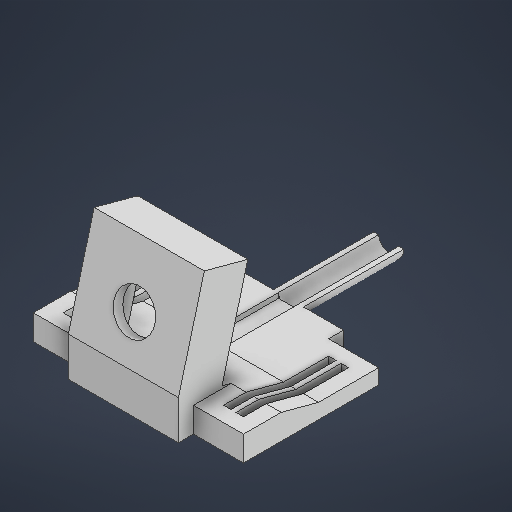
# Autodesk Inventor part: pieza prueba autodesk
Saved by Autodesk Inventor 2027.1 (Build 311270010, 270A)
## iProperties
Created: 2026-09-10
Part Number: pieza prueba autodesk
Material: Genérico
Document SubType Name: Modeling
Designer: marco
Density: 1 g/cm^3
Appearance: Valor por defecto
Author: marco
Autodesk Inventor part; units mm, degrees
ref_plane "YZ Plane" through (0, 0, 0) normal (1, 0, 0) x (0, 1, 0)
ref_plane "XZ Plane" through (0, 0, 0) normal (0, 1, 0) x (-1, 0, 0)
ref_plane "XY Plane" through (0, 0, 0) normal (0, 0, 1) x (1, 0, 0)
sketch "Boceto9" plane through (0, 0, 0) normal (1, 0, 0) x (0, 1, 0)
  line L0 (0, 0) -> (0, -3)
  line L1 (0, -3) -> (0, -33)
  line L2 (0, -3) -> (3, -3)
  line L3 (3, -3) -> (3, -33)
  line L4 (3, -33) -> (0, -33)
  line L5 (3, -3) -> (3, -18)
  line L6 (3, -18) -> (7.8231, 0)
  line L7 (7.8231, 0) -> (0, 0)
  dimension "d22" = 3
  dimension "d23" = 30
  dimension "d24" = 3
  dimension "d25" = 15
  dimension "d26" = 15
  constraints: 16 end point, 3 perpendicular, 1 horizontal, 1 midpoint, 1 point on line, 1 vertical
  measures "d22" distance of L0.start L0.end
  measures "d23" distance of L0.end L1.end
  measures "d24" distance of L0.end L2.end
  measures "d25" distance of L2.end L5.end
  measures "d26" angle of L6 L5
extrude "Extrusión6" add sketch "Boceto9" along normal blind 22
sketch "Boceto10" plane through (0, 0, -33) normal (0, -1, 0) x (1, 0, 0)
  line L0 (22, 15) -> (22, 33) projected
  line L1 (22, 33) -> (22, 30)
  line L2 (22, 30) -> (22.6923, 30)
  line L3 (22, 30) -> (32, 30)
  line L4 (32, 30) -> (32, 3)
  line L5 (32, 3) -> (22, 3)
  line L6 (22, 0) -> (22, 15) projected
  line L7 (0, 33) -> (22, 33) projected
  line L8 (11, 33) -> (11, 0)
  line L9 (0, 0) -> (22, 0) projected
  line L10 (0, 15) -> (0, 33)
  line L11 (0, 33) -> (0, 30)
  line L12 (0, 30) -> (-0.6923, 30)
  line L13 (0, 30) -> (-10, 30)
  line L14 (-10, 30) -> (-10, 3)
  line L15 (-10, 3) -> (0, 3)
  line L16 (0, 0) -> (0, 15)
  line L17 (22, 33) -> (0, 33)
  line L18 (22, 0) -> (0, 0)
  dimension "d29" = 3
  dimension "d31" = 10
  dimension "d32" = 27
  constraints: 30 end point, 10 symmetric about line, 4 point on line, 3 perpendicular, 2 midpoint, 1 horizontal
  measures "d29" distance of L0.end L1.end
  measures "d31" distance of L1.end L3.end
  measures "d32" distance of L3.end L4.end
extrude "Extrusión7" add sketch "Boceto10" against normal blind 5 contours L0 L2 L3 L4 L5 L6 | L10 L16 L15 L14 L13 L12
sketch "Boceto11" plane through (32, 0, -3) normal (1, 0, 0) x (0, 0, -1)
  line L0 (27, 3) -> (15, 3) projected
  line L1 (15, 3) -> (7.5359, 5) projected
  line L2 (27, 5) -> (7.5359, 5) projected
  line L3 (27, 3) -> (15, 3) projected
  line L4 (15, 3) -> (7.5359, 5) projected
  line L5 (27, 5) -> (7.5359, 5) projected
  line L6 (27, 3) -> (27, 5) projected
  line L7 (27, 0) -> (0, 0) projected
  line L8 (0, 5) -> (27, 5) projected
  line L9 (0, 5) -> (27, 5) projected
  line L10 (27, 5) -> (7.5359, 5) projected
  line L11 (0, 5) -> (7.5359, 5) projected
  line L12 (27, 0) -> (0, 0) projected
  line L13 (27, 0) -> (27, 5) projected
  line L14 (0, 5) -> (27, 5) projected
  line L15 (0, 0) -> (0, 5) projected
  line L16 (27, 0) -> (30, 0) projected
  line L17 (30, 0) -> (30, 3) projected
  line L18 (27, 0) -> (27, 3) projected
  line L19 (30, 3) -> (27, 3) projected
  line L20 (30, 0) -> (30, 3) projected
  line L21 (27, 0) -> (30, 0) projected
  line L22 (30, 0) -> (30, 3) projected
  line L23 (30, 0) -> (30, 3) projected
  line L24 (30, 3) -> (27, 3) projected
  line L25 (30, 3) -> (27, 3) projected
  line L26 (27, 3) -> (15, 3) projected
  line L27 (27, 3) -> (15, 3) projected
  line L28 (30, 3) -> (27, 3) projected
  line L29 (-3, 0) -> (0, 0) projected
  line L30 (0, 0) -> (27, 0) projected
  line L31 (27, 0) -> (30, 0) projected
  line L32 (27, 0) -> (30, 0) projected
  line L33 (27, 0) -> (0, 0) projected
  line L34 (-3, 0) -> (0, 0) projected
  line L35 (15, 3) -> (7.5359, 5) projected
  line L36 (7.5359, 5) -> (-3, 7.8231) projected
  line L37 (7.5359, 5) -> (-3, 7.8231) projected
  line L38 (15, 3) -> (7.5359, 5) projected
  line L39 (27, 0) -> (27, 3) projected
  line L40 (27, 0) -> (27, 5) projected
  line L41 (15, 3) -> (7.5359, 5) projected
  line L42 (7.5359, 5) -> (27, 5) projected
  line L43 (27, 3) -> (27, 5) projected
  line L44 (27, 3) -> (15, 3) projected
  line L45 (27, 3) -> (15, 3) projected
  line L46 (27, 3) -> (27, 5) projected
  line L47 (7.5359, 5) -> (27, 5) projected
  line L48 (15, 3) -> (7.5359, 5) projected
  line L49 (27, 0) -> (27, 5) projected
  line L50 (27, 3) -> (27, 5) projected
  line L51 (27, 0) -> (27, 3) projected
  line L52 (27, 5) -> (0, 5) projected
  line L53 (7.5359, 5) -> (0, 5) projected
  line L54 (7.5359, 5) -> (27, 5) projected
  line L55 (0, 0) -> (27, 0) projected
  line L56 (0, 0) -> (0, 5) projected
  line L57 (27, 5) -> (0, 5) projected
  line L58 (27, 0) -> (27, 5) projected
  line L59 (0, 0) -> (27, 0) projected
  line L60 (27, 5) -> (0, 5) projected
  line L61 (27, 3) -> (27, 0) projected
  line L62 (27, 3) -> (27, 5) projected
  line L63 (30, 3) -> (27, 3) projected
  line L64 (30, 0) -> (30, 3) projected
  line L65 (27, 0) -> (30, 0) projected
  line L66 (27, 0) -> (27, 5) projected
  line L67 (27, 3) -> (27, 0) projected
  line L68 (27, 3) -> (27, 5) projected
  line L69 (27, 0) -> (27, 5) projected
  line L70 (27, 3) -> (27, 0) projected
  line L71 (27, 0) -> (30, 0) projected
  line L72 (30, 0) -> (30, 3) projected
  line L73 (30, 3) -> (27, 3) projected
  constraints: 14 other
extrude "Extrusión8" cut sketch "Boceto11" against normal up to surface (42 mm away) contours L0 L1 L2 L6
sketch "Boceto12" plane through (22, 0, 0) normal (1, 0, 0) x (0, 0, -1)
  line L0 (10.5359, 5) -> (0, 7.8231) projected
  line L1 (0, 7.8231) -> (5.1764, 27.1416)
  line L2 (0, 7.8231) -> (20, 7.8231) construction
  line L3 (5.1764, 27.1416) -> (13.8697, 24.8122)
  line L4 (13.8697, 24.8122) -> (8.6933, 5.4937)
  point P0 (0, 0)
  dimension "d37" = 20
  dimension "d38" = 75
  dimension "d40" = 9
  constraints: 8 end point, 2 perpendicular, 1 equal length, 1 horizontal, 1 point on line
  measures "d37" distance of L0.end L1.end
  measures "d38" angle of L2 L1
  measures "d40" distance of L1.end L3.end
extrude "Extrusión9" add sketch "Boceto12" against normal up to surface (22 mm away)
sketch "Boceto13" plane through (22, 24.8122, -13.8697) normal (0, -0.2588, -0.9659) x (-1, 0, 0)
  line L0 (22, -20) -> (0, -20) projected
  line L1 (0, -20) -> (3, -20)
  line L2 (0, 0) -> (0, -20) projected
  line L3 (0, 0) -> (3, 0)
  line L4 (0, 0) -> (22, 0) projected
  line L5 (3, 0) -> (3, -16.1177)
  line L6 (0, 0) -> (0, -3)
  line L7 (0, -3) -> (22, -3)
  line L8 (22, -3) -> (22, 0)
  line L9 (22, 0) -> (19, 0)
  line L10 (19, 0) -> (19, -20)
  line L11 (3, -3) -> (3, -20)
  point P0 (22, -27.5565)
  point P1 (19, -3)
  dimension "d43" = 3
  dimension "d44" = 3
  dimension "d45" = 3
  dimension "d46" = 3
  constraints: 18 end point, 7 point on line, 4 perpendicular, 1 vertical
  measures "d43" distance of L0.end L1.end
  measures "d44" distance of L2.start L3.end
  measures "d45" distance of L2.start L6.end
  measures "d46" distance of L8.end L9.end
extrude "Extrusión10" cut sketch "Boceto13" against normal blind 7 contours L0 L11 L5 L7 L10
sketch "Boceto14" plane through (0, 0, -33) normal (0, -1, 0) x (1, 0, 0)
  line L0 (32, 30) -> (32, 22.4641) projected
  line L1 (32, 30) -> (32, 27)
  line L2 (32, 30) -> (29, 30)
  line L3 (22, 30) -> (32, 30) projected
  line L4 (29, 30) -> (29, 3)
  line L5 (32, 3) -> (32, 30) projected
  line L6 (29, 3) -> (32, 3)
  line L7 (32, 3) -> (32, 6)
  line L8 (32, 6) -> (25, 6)
  line L9 (25, 6) -> (22, 6)
  line L10 (22, 6) -> (22, 30)
  line L11 (22, 30) -> (22, 27)
  line L12 (22, 27) -> (32, 27)
  line L13 (22, 3) -> (25, 3)
  line L14 (25, 3) -> (25, 30)
  line L15 (29, 27) -> (27.5, 27)
  line L16 (27.5, 27) -> (27.5, 6)
  line L17 (27.5, 6) -> (29, 6)
  line L18 (29, 6) -> (29, 27)
  line L19 (25, 27) -> (26.5, 27)
  line L20 (26.5, 27) -> (26.5, 6)
  line L21 (26.5, 6) -> (25, 6)
  line L22 (25, 6) -> (25, 27)
  line L23 (0, 33) -> (22, 33) projected
  line L24 (11, 33) -> (11, -0.1638)
  line L25 (-10, 30) -> (-10, 22.4641)
  line L26 (-10, 30) -> (-10, 27)
  line L27 (-10, 30) -> (-7, 30)
  line L28 (0, 30) -> (-10, 30)
  line L29 (-7, 30) -> (-7, 3)
  line L30 (-10, 3) -> (-10, 30)
  line L31 (-7, 3) -> (-10, 3)
  line L32 (-10, 3) -> (-10, 6)
  line L33 (-10, 6) -> (-3, 6)
  line L34 (-3, 6) -> (0, 6)
  line L35 (0, 6) -> (0, 30)
  line L36 (0, 30) -> (0, 27)
  line L37 (0, 27) -> (-10, 27)
  line L38 (0, 3) -> (-3, 3)
  line L39 (-3, 3) -> (-3, 30)
  line L40 (-7, 27) -> (-5.5, 27)
  line L41 (-5.5, 27) -> (-5.5, 6)
  line L42 (-5.5, 6) -> (-7, 6)
  line L43 (-7, 6) -> (-7, 27)
  line L44 (-3, 27) -> (-4.5, 27)
  line L45 (-4.5, 27) -> (-4.5, 6)
  line L46 (-4.5, 6) -> (-3, 6)
  line L47 (-3, 6) -> (-3, 27)
  line L48 (22, 33) -> (0, 33)
  point P0 (-7, 6)
  point P1 (25, 6)
  point P2 (29, 6)
  dimension "d52" = 3
  dimension "d53" = 3
  dimension "d54" = 3
  dimension "d55" = 7
  dimension "d56" = 90
  dimension "d57" = 3
  dimension "d58" = 3
  dimension "d59" = 3
  dimension "d60" = 1.5
  dimension "d61" = 1.5
  dimension "d62" = 21
  constraints: 90 end point, 26 point on line, 25 symmetric about line, 7 perpendicular, 4 parallel, 3 horizontal, 1 midpoint, 1 vertical
  measures "d52" distance of L0.start L1.end
  measures "d53" distance of L0.start L2.end
  measures "d54" distance of L5.start L7.end
  measures "d55" distance of L7.end L8.end
  measures "d56" angle of L8 L7
  measures "d57" distance of L8.end L9.end
  measures "d58" distance of L10.end L11.end
  measures "d59" distance of L13.start L13.end
  measures "d60" distance of L17.end L16.end
  measures "d61" distance of L20.end L21.end
  measures "d62" distance of L19.end L20.end
extrude "Extrusión11" cut sketch "Boceto14" against normal blind 7 contours L4 L8 L16 L12 | L12 L20 L8 L14 | L37 L41 L33 L29 | L39 L33 L45 L37
sketch "Boceto15" plane through (22, 26.624, -7.1082) normal (0, -0.2588, -0.9659) x (-1, 0, 0)
  line L0 (19, -20) -> (3, -20) projected
  line L1 (19, -3) -> (19, -20) projected
  line L2 (3, -3) -> (19, -3) projected
  line L3 (3, -20) -> (3, -3) projected
  line L4 (22, -19.0155) -> (0, -19.0155) projected
  line L5 (3, -20) -> (19, -20)
  line L6 (25, -20) -> (-3, -20) projected
  line L7 (3, -20) -> (11, -20)
  line L8 (3, -20) -> (19, -20)
  line L9 (11, -20) -> (11, -3)
  line L10 (11, -20) -> (11, -11.5)
  circle A0 centre (11, -11.5) radius 4.1
  point P0 (22, -27.5565)
  dimension "d65" = 8.5
  dimension "d66" = 8.2
  constraints: 10 end point, 2 midpoint, 1 centre point, 1 coincident, 1 collinear, 1 horizontal
  measures "d65" distance of L7.end L10.end
  measures "d66" diameter of A0
extrude "Extrusión12" cut sketch "Boceto15" against normal blind 2 contours A0 L9 | L9 A0
sketch "Boceto17" plane through (22, 24.8122, -13.8697) normal (0, -0.2588, -0.9659) x (-1, 0, 0)
  line L0 (0, 0) -> (1.5, 0)
  line L1 (0, 0) -> (22, 0) projected
  line L2 (1.5, 0) -> (1.5, -1.5)
  line L3 (22, 0) -> (20.5, 0)
  line L4 (20.5, 0) -> (20.5, -1.5)
  line L5 (0, -20) -> (1.5, -20)
  line L6 (3, -20) -> (0, -20) projected
  line L7 (1.5, -20) -> (1.5, -18.5)
  line L8 (1.5, -18.5) -> (20.5, -18.5)
  circle A0 centre (1.5, -18.5) radius 0.75
  circle A1 centre (20.5, -18.5) radius 0.75
  circle A2 centre (20.5, -1.5) radius 0.75
  circle A3 centre (1.5, -1.5) radius 0.75
  point P0 (22, -27.5565)
  dimension "d69" = 1.5
  dimension "d70" = 1.5
  dimension "d71" = 1.5
  dimension "d72" = 1.5
  dimension "d73" = 1.5
  dimension "d74" = 1.5
  dimension "d75" = 19
  dimension "d76" = 1.5
  dimension "d77" = 1.5
  dimension "d78" = 1.5
  dimension "d79" = 1.5
  constraints: 14 end point, 4 centre point, 4 coincident, 4 perpendicular, 2 point on line, 1 midpoint
  measures "d69" distance of L0.start L0.end
  measures "d70" distance of L0.end L2.end
  measures "d71" distance of L1.end L3.end
  measures "d72" distance of L3.end L4.end
  measures "d73" distance of L5.start L5.end
  measures "d74" distance of L5.end L7.end
  measures "d75" distance of L7.end L8.end
  measures "d76" diameter of A0
  measures "d77" diameter of A1
  measures "d78" diameter of A2
  measures "d79" diameter of A3
extrude "Extrusión13" cut sketch "Boceto17" against normal blind 2
sketch "Boceto18" plane through (3, 7.3054, -1.9319) normal (0, 0.9659, -0.2588) x (1, 0, 0)
  line L0 (19, 8.9076) -> (19, 7) projected
  line L1 (19, 8.9076) -> (19, 16.635)
  line L2 (-6, 16.635) -> (22, 16.635) projected
  line L3 (19, 16.635) -> (-3, 16.635)
  line L4 (-3, 16.635) -> (8, 16.635)
  line L5 (8, 16.635) -> (6, 16.635)
  line L6 (6, 16.635) -> (10, 16.635)
  line L7 (10, 16.635) -> (10, 0.0248)
  line L8 (10, 0.0248) -> (6, 0.0248)
  line L9 (6, 0.0248) -> (6, 16.635)
  point P0 (-3, 0.0248)
  dimension "d82" = 2
  dimension "d83" = 4
  dimension "d84" = 4
  constraints: 16 end point, 3 point on line, 2 perpendicular, 1 horizontal, 1 midpoint, 1 vertical
  measures "d82" distance of L4.end L5.end
  measures "d83" distance of L5.end L6.end
  measures "d84" distance of L7.end L8.end
extrude "Extrusión14" cut sketch "Boceto18" against normal blind 1
sketch "Boceto19" plane through (0, 3, -33) normal (0, 1, 0) x (1, 0, 0)
  line L0 (0, 0) -> (22, 0) projected
  line L1 (9, -15) -> (9, 0)
  line L2 (9, 0) -> (13, 0)
  line L3 (13, 0) -> (13, -15)
  line L4 (13, -15) -> (25, -15) projected
  line L5 (13, -15) -> (13, -17.039)
  line L6 (13, -15) -> (13, -31.0442) projected
  line L7 (9, -31.303) -> (9, -15.2588) projected
  line L8 (9, -17.039) -> (13, -17.039)
  line L9 (9, -17.039) -> (9, -14.1278)
  point P0 (0, -33)
  dimension "d87" = 4
  constraints: 12 end point, 4 point on line, 1 parallel, 1 perpendicular
  measures "d87" distance of L1.end L2.end
extrude "Extrusión16" cut sketch "Boceto19" against normal blind 1
sketch "Boceto20" plane through (0, 0, -33) normal (0, 0, -1) x (-1, 0, 0)
  line L0 (-13, 2) -> (-9, 2) projected
  line L1 (-11, 2) -> (-9, 2)
  line L2 (-13, 2) -> (-13, 3) projected
  line L3 (-13, 3) -> (-11, 3)
  circle A0 centre (-11, 3) radius 3
  circle A1 centre (-11, 3) radius 2
  line L4 (-13, 3) -> (-22, 3) projected
  line L5 (-14.8156, 3) -> (-7.3833, 3)
  point P0 (0, 0)
  point P1 (-8, 3)
  point P2 (-9, 3)
  point P3 (-12.7321, 2)
  point P4 (-14, 3)
  dimension "d92" = 2
  dimension "d93" = 6
  dimension "d94" = 4
  constraints: 6 end point, 2 centre point, 2 coincident, 2 collinear, 1 horizontal, 1 midpoint, 1 point on line
  measures "d92" distance of L2.end L3.end
  measures "d93" diameter of A0
  measures "d94" diameter of A1
extrude "Extrusión17" add sketch "Boceto20" along normal blind 20 contours L0 A1 L5 A0 L4 L2
